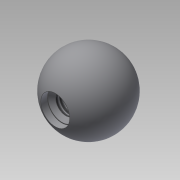
# Autodesk Inventor part: Ручка
Saved by Autodesk Inventor 2014 SP1 (Build 180222100, 222)
## iProperties
Created: 2021-12-02
Part Number: Ручка
Material: Типовые
Document SubType Name: Modeling
Designer: Украинцев
Mass: 12.899 g
Surface Area: 32.8234 cm^2
Volume: 12.899 cm^3
Density: 1 g/cm^3
Appearance: По умолчанию
Author: Украинцев
Autodesk Inventor part; units mm, degrees
ref_plane "YZ Plane" through (0, 0, 0) normal (1, 0, 0) x (0, 1, 0)
ref_plane "XZ Plane" through (0, 0, 0) normal (0, 1, 0) x (-1, 0, 0)
ref_plane "XY Plane" through (0, 0, 0) normal (0, 0, 1) x (1, 0, 0)
sketch "Эскиз1" plane through (0, 0, 0) normal (0, 0, 1) x (1, 0, 0)
  arc A0 (0, 0) -> (0, 30) centre (0, 15) ccw
  line L0 (0, 0) -> (0, 30)
  dimension "d0" = 30
  constraints: 2 end point, 2 point on circle, 1 centre point, 1 vertical, 1 vertical alignment
  measures "d0" diameter of A0
revolve "Вращение1" add sketch "Эскиз1" angle 360 about axis through (0, 0, 0) along (0, 1, 0)
sketch "Эскиз2" plane through (0, 0, 0) normal (0, 1, 0) x (-1, 0, 0)
  point P0 (0, 0)
  point P1 (0, 0)
  constraints: 1 coincident
hole "Отверстие1" at (0, 0, 0) direction (0, 1, 0) diameter 8.376 depth 18 tip angle 118 counterbore diameter 12 counterbore depth 4 thread size "M10x1.5" class "6H" standard "ISO Metric profile"
chamfer "Фаска1" distance 1.6 angle 45 1 edges at (0, 4, 4.188)
